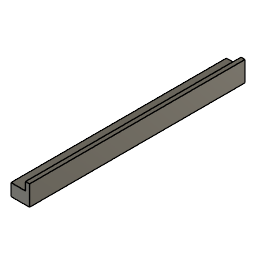
cover rolls mount right part 2 (Autodesk Fusion 360 design; units mm, degrees)
Autodesk Fusion 360 part; units mm, degrees
sketch "Szkic1" plane through (0, 0, 0) normal (0, 0, 1) x (1, 0, 0)
  line L0 (45, 135) -> (-35, 135)
  line L1 (-35, 135) -> (-35, -130)
  line L2 (-35, -130) -> (45, -130)
  circle A0 centre (25, -120) radius 1.75
  circle A1 centre (-25, -120) radius 1.75
  circle A2 centre (-25, -70) radius 1.75
  circle A3 centre (-25, -20) radius 1.75
  circle A4 centre (-25, 30) radius 1.75
  circle A5 centre (-25, 80) radius 1.75
  circle A6 centre (-15, 125) radius 3.5
  circle A7 centre (20, 125) radius 3.5
  circle A8 centre (20, 105) radius 3.5
  circle A9 centre (-15, 105) radius 3.5
  line L3 (45, -130) -> (45, -105)
  line L4 (45, -105) -> (-35, -105)
  line L5 (-35, -105) -> (-35, -130)
  line L6 (-35, -130) -> (45, -130)
  line L7 (-35, -130) -> (-17, -130)
  line L8 (-17, -130) -> (-17, 135)
  line L9 (-17, 135) -> (-35, 135)
  line L10 (-35, 135) -> (-35, -130)
  line L11 (-17, 135) -> (-17, -130)
  line L12 (-17, -130) -> (-12, -130)
  line L13 (-12, -130) -> (-12, 135)
  line L14 (-12, 135) -> (-17, 135)
  dimension "d1" = 5
  constraint perpendicular L3 L4
  constraint parallel L3 L5
  constraint parallel L4 L6
  constraint perpendicular L2 L3
  constraint perpendicular L7 L8
  constraint parallel L7 L9
  constraint parallel L8 L10
  constraint perpendicular L1 L7
  constraint perpendicular L11 L12
  constraint parallel L11 L13
  constraint parallel L12 L14
  measures "d1" distance of L8.end L13.end
extrude "Wyciągnięcie proste1" add sketch "Szkic1" along normal blind 25 contours L0 A6 L8 L11 L13 L14 | A6 L8 L11 L13 | A6 A9 L8 L11 L13 | A9 L8 L11 L13 | A9 L4 L8 L11 L13
extrude "Wyciągnięcie proste2" add sketch "Szkic1" along normal blind 15 contours L0 L1 A6 A9 L4 L8 L9 L10 L11 | A6 L8 L11 | A9 L8 L11
extrude "Wyciągnięcie proste3" add 1 faces at (-21.3333, -105, 5) along direction (0, -1, 0) blind 26
extrude "Wyciągnięcie proste4" cut sketch "Szkic1" along normal blind 37 contours A1
sketch "Szkic2" plane through (0, 0, 0) normal (0, 0, -1) x (1, 0, 0)
  circle A0 centre (-25, 120) radius 1.75
  circle A1 centre (-25, -30) radius 1.75
  circle A2 centre (-25, -80) radius 1.75
  circle A3 centre (-25, 20) radius 1.75
  circle A4 centre (-25, 70) radius 1.75
  line L0 (-12, -135) -> (-12, 131)
  line L1 (-12, 131) -> (-35, 131)
  line L2 (-35, 131) -> (-35, -135)
  line L3 (-35, -135) -> (-12, -135)
  circle A5 centre (-25, 120) radius 2
  circle A6 centre (-25, 120) radius 3.5
  circle A7 centre (-25, 70) radius 2
  circle A8 centre (-25, 20) radius 2
  circle A9 centre (-25, -30) radius 2
  circle A10 centre (-25, -80) radius 2
  dimension "d10" = 4
  dimension "d11" = 7
  dimension "d12" = 4
  dimension "d13" = 4
  dimension "d14" = 4
  dimension "d15" = 4
  constraint concentric A0 A5
  constraint concentric A0 A6
  constraint concentric A4 A7
  constraint concentric A3 A8
  constraint concentric A1 A9
  constraint concentric A2 A10
  measures "d10" diameter of A5
  measures "d11" diameter of A6
  measures "d12" diameter of A7
  measures "d13" diameter of A8
  measures "d14" diameter of A9
  measures "d15" diameter of A10
extrude "Wyciągnięcie proste5" cut sketch "Szkic2" against normal blind 100 contours A5 | A7 | A8 | A9 | A10
extrude "Wyciągnięcie proste6" cut sketch "Szkic2" against normal blind 4 contours A6
